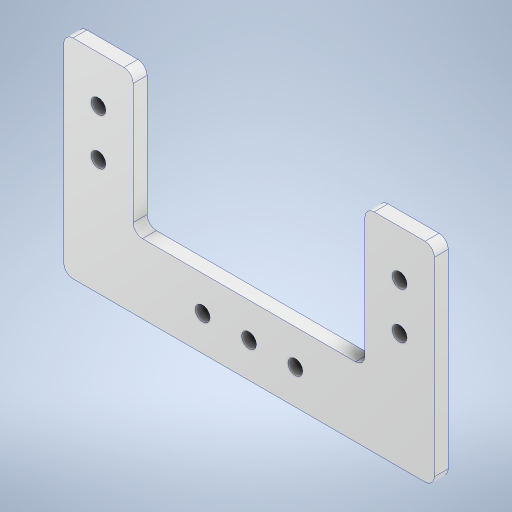
# Autodesk Inventor part: 射出_固定6
Saved by Autodesk Inventor 2023 (Build 270158000, 158)
## iProperties
Created: 2022-04-20
Part Number: 射出_固定6
Material: アルミニウム 6061
Document SubType Name: Modeling
Designer: yuta
Density: 2.7 g/cm^3
Appearance: アルミニウム - フラット
Author: yuta
Autodesk Inventor part; units mm, degrees
ref_plane "YZ Plane" through (0, 0, 0) normal (1, 0, 0) x (0, 1, 0)
ref_plane "XZ Plane" through (0, 0, 0) normal (0, 1, 0) x (-1, 0, 0)
ref_plane "XY Plane" through (0, 0, 0) normal (0, 0, 1) x (1, 0, 0)
sketch "スケッチ1" plane through (0, 0, 0) normal (0, 0, 1) x (1, 0, 0)
  line L0 (0, 0) -> (80, 0)
  line L1 (80, 0) -> (80, 45)
  line L2 (80, 45) -> (0, 45)
  line L3 (0, 45) -> (0, 0)
  dimension "d0" = 80
  dimension "d1" = 45
  constraints: 8 end point, 2 parallel, 1 horizontal, 1 perpendicular
  measures "d0" distance of L2.end L1.end
  measures "d1" distance of L1.end L0.end
extrude "押し出し1" add sketch "スケッチ1" along normal blind 3
sketch "スケッチ2" plane through (0, 0, 3) normal (0, 0, 1) x (1, 0, 0)
  line L0 (0, 45) -> (0, 0) projected
  line L1 (0, 0) -> (80, 0) projected
  line L2 (80, 45) -> (0, 45) projected
  line L3 (40, 45) -> (40, 0) construction
  point P0 (7.5, 35)
  point P1 (7.5, 25)
  point P2 (30, 7.5)
  point P3 (72.5, 35)
  point P4 (72.5, 25)
  point P5 (50, 7.5)
  point P6 (40, 7.5)
  dimension "d4" = 7.5
  dimension "d5" = 35
  dimension "d6" = 10
  dimension "d7" = 7.5
  dimension "d8" = 7.5
  dimension "d9" = 30
  constraints: 3 symmetric about line, 2 end point, 2 midpoint, 1 point on line
  measures "d4" distance from line of L0 point (7.5, 35)
  measures "d5" distance from line of L1 point (7.5, 35)
  measures "d6" distance of point (7.5, 25) point (7.5, 35)
  measures "d7" distance from line of L0 point (7.5, 25)
  measures "d8" distance from line of L1 point (30, 7.5)
  measures "d9" distance from line of L0 point (30, 7.5)
hole "穴1" at (7.5, 35, 3) at (7.5, 25, 3) at (30, 7.5, 3) at (72.5, 35, 3) at (72.5, 25, 3) at (50, 7.5, 3) at (40, 7.5, 3) direction (0, 0, -1) diameter 3.2 end through all
sketch "スケッチ3" plane through (0, 0, 3) normal (0, 0, 1) x (1, 0, 0)
  line L0 (80, 45) -> (0, 45) projected
  line L1 (15, 45) -> (65, 45)
  line L2 (65, 45) -> (65, 15)
  line L3 (65, 15) -> (15, 15)
  line L4 (15, 15) -> (15, 45)
  line L5 (0, 45) -> (0, 0) projected
  line L6 (0, 0) -> (80, 0) projected
  dimension "d17" = 50
  dimension "d18" = 30
  dimension "d19" = 15
  dimension "d20" = 15
  constraints: 8 end point, 2 parallel, 1 horizontal, 1 perpendicular, 1 point on line
  measures "d17" distance of L2.end L3.end
  measures "d18" distance of L1.end L2.end
  measures "d19" distance between parallel lines of L5 L4
  measures "d20" distance between parallel lines of L6 L3
extrude "押し出し2" cut sketch "スケッチ3" against normal blind 3
fillet "フィレット1" radius 2 8 edges at (15, 45, 1.5) (65, 15, 1.5) (65, 45, 1.5) (80, 45, 1.5) (0, 45, 1.5) (0, 0, 1.5) (80, 0, 1.5) (15, 15, 1.5)
